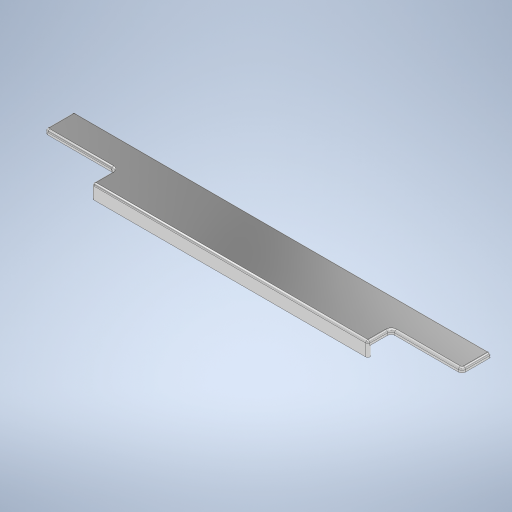
# Autodesk Inventor part: Häfele Alu profile 126.26.201 295 mm Chrome polished
Saved by Autodesk Inventor 2024 (Build 280153000, 153)
## iProperties
Created: 2019-10-03
Part Number: Häfele Alu profile 126.26.201 295 mm Chrome polished
Material: Aluminum 6061
Document SubType Name: Modeling
Designer: RokasM
Density: 2.7 g/cm^3
Appearance: Chrome - Polished
Author: RokasM
Autodesk Inventor part; units mm, degrees
ref_plane "YZ Plane" through (0, 0, 0) normal (1, 0, 0) x (0, 1, 0)
ref_plane "XZ Plane" through (0, 0, 0) normal (0, 1, 0) x (-1, 0, 0)
ref_plane "XY Plane" through (0, 0, 0) normal (0, 0, 1) x (1, 0, 0)
sketch "Sketch1" plane through (0, 0, 0) normal (1, 0, 0) x (0, 1, 0)
  line L0 (-37, -7) -> (-37, 3)
  line L1 (-37, 3) -> (0, 3)
  line L2 (0, 3) -> (0, 0)
  line L3 (0, 0) -> (-34, 0)
  line L4 (-34, 0) -> (-34, -7)
  line L5 (-34, -7) -> (-37, -7)
  dimension "d0" = 37
  dimension "d1" = 10
  dimension "d2" = 3
  constraints: 12 end point, 6 perpendicular, 2 coincident, 1 vertical
  measures "d0" distance between parallel lines of L2 L0
  measures "d1" distance between parallel lines of L5 L1
  measures "d2" distance between parallel lines of L3 L1
extrude "handle_ex" add sketch "Sketch1" along normal mid plane 295
sketch "Sketch2" plane through (-147.5, -37, 3) normal (0, 0, 1) x (1, 0, 0)
  line L0 (245, 16.5) -> (295, 16.5)
  line L1 (295, 16.5) -> (295, 0)
  line L2 (295, 0) -> (245, 0)
  line L3 (245, 0) -> (245, 16.5)
  line L4 (0, 0) -> (295, 0) projected
  line L5 (295, 37) -> (295, 0) projected
  point P0 (147.5, 37)
  dimension "d5" = 50
  dimension "d6" = 16.5
  constraints: 8 end point, 2 collinear, 2 parallel, 1 horizontal, 1 perpendicular
  measures "d5" distance of L1.end L2.end
  measures "d6" distance of L0.end L1.end
extrude "handle_cutouts" cut sketch "Sketch2" against normal through all
mirror "handle_cutouts_mirror" about plane through (0, 0, 0) normal (1, 0, 0) of "handle_cutouts"
sketch "Sketch3" plane through (0, 0, 0) normal (1, 0, 0) x (0, 1, 0)
  line L0 (-11, -8) -> (-11.5, -6.5)
  line L1 (-11.5, -6.5) -> (-11, -6.5)
  line L2 (-11, -6.5) -> (-11.5, -5)
  line L3 (-11.5, -5) -> (-11, -5)
  line L4 (-11, -5) -> (-11.5, -3.5)
  line L5 (-11.5, -3.5) -> (-11, -3.5)
  line L6 (-11, -3.5) -> (-11.5, -2)
  line L7 (-11.5, -2) -> (-11, -2)
  line L8 (-11, -2) -> (-11, 0)
  line L9 (-11, 0) -> (-9, 0)
  line L10 (-9, 0) -> (-9, -2)
  line L11 (-9, -2) -> (-8.5, -2)
  line L12 (-8.5, -2) -> (-9, -3.5)
  line L13 (-9, -3.5) -> (-8.5, -3.5)
  line L14 (-8.5, -3.5) -> (-9, -5)
  line L15 (-9, -5) -> (-8.5, -5)
  line L16 (-8.5, -5) -> (-9, -6.5)
  line L17 (-9, -6.5) -> (-8.5, -6.5)
  line L18 (-8.5, -6.5) -> (-9, -8)
  line L19 (-9, -8) -> (-11, -8)
  line L20 (-20.5, 0) -> (0, 0) projected
  line L21 (0, 0) -> (0, 3) projected
  dimension "d9" = 0.5
  dimension "d11" = 1.5
  dimension "d12" = 2
  dimension "d13" = 2
  dimension "d14" = 8
  dimension "d15" = 8.5
  constraints: 40 end point, 14 equal length, 8 parallel, 6 collinear, 2 perpendicular
  measures "d9" distance of L6.end L7.end
  measures "d11" distance between parallel lines of L5 L7
  measures "d12" distance of L18.end L0.start
  measures "d13" distance of L8.end L9.end
  measures "d14" distance between parallel lines of L19 L9
  measures "d15" distance from line of L21 L17.end
extrude "harpoon_wedge" add sketch "Sketch3" along normal mid plane 224
fillet "fillet" radius 2.5 4 edges at (97.5, -20.5, 1.5) (147.5, -20.5, 1.5) (-97.5, -20.5, 1.5) (-147.5, -20.5, 1.5)
fillet "fillet" radius 1.5 11 edges at (-147.5, -10.25, 3) (-122.5, -20.5, 3) (-97.5, -28.75, 3) (0, -37, 3) (-97.5, -37, -2) (-97.5, -34, -3.5) (97.5, -28.75, 3) (97.5, -37, -2) (97.5, -34, -3.5) (122.5, -20.5, 3) (147.5, -10.25, 3)
fillet "fillet" radius 1 3 edges at (147.5, 0, 1.5) (0, 0, 3) (-147.5, 0, 1.5)
sketch "Sketch4" plane through (0, 0, 0) normal (1, 0, 0) x (0, 1, 0)
  line L0 (-11.5, 0) -> (-8.5, 0)
  line L1 (-8.5, 0) -> (-8.5, -8)
  line L2 (-8.5, -8) -> (-11.5, -8)
  line L3 (-11.5, -8) -> (-11.5, 0)
  line L4 (-11, -8) -> (-9, -8) projected
  point P0 (0, 0)
  point P1 (-10, -8)
  point P2 (-10, -8)
  dimension "d21" = 3
  dimension "d22" = 8
  constraints: 8 end point, 2 midpoint, 2 parallel, 1 coincident, 1 collinear, 1 horizontal, 1 perpendicular
  measures "d21" distance of L1.end L2.end
  measures "d22" distance of L0.end L1.end
extrude "cut_body" add sketch "Sketch4" along normal mid plane 224 separate body
equation "\"d3\" = Length"
equation "\"d23\" = d16"
equation "\"Length\" = 295"
equation "\"d16\" = 224"
